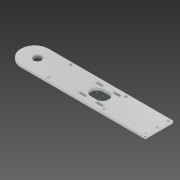
# Autodesk Inventor part: bovenarm - links
Saved by Autodesk Inventor 2020 (Build 240168000, 168)
## iProperties
Created: 2020-05-18
Part Number: bovenarm - links
Material: Generic
Document SubType Name: Modeling
Designer: stefa
Density: 1 g/cm^3
Appearance: Aluminum - Polished
Author: stefa
Autodesk Inventor part; units mm, degrees
ref_plane "YZ Plane" through (0, 0, 0) normal (1, 0, 0) x (0, 1, 0)
ref_plane "XZ Plane" through (0, 0, 0) normal (0, 1, 0) x (-1, 0, 0)
ref_plane "XY Plane" through (0, 0, 0) normal (0, 0, 1) x (1, 0, 0)
sketch "Sketch1" plane through (0, 0, 0) normal (0, 1, 0) x (-1, 0, 0)
  line L0 (0, 0) -> (250, 0)
  line L1 (250, 0) -> (250, -50)
  line L2 (250, -50) -> (0, -50)
  line L3 (0, -50) -> (0, 0)
  circle A0 centre (220, -25) radius 7
  line L4 (112.355, -25) -> (102.355, -25) construction
  line L5 (112.355, -13.9) -> (102.355, -13.9)
  line L6 (102.355, -36.1) -> (112.355, -36.1)
  arc A1 (112.355, -36.1) -> (112.355, -13.9) centre (112.355, -25) ccw
  arc A2 (102.355, -13.9) -> (102.355, -36.1) centre (102.355, -25) ccw
  line L7 (127.855, -40.5) -> (117.855, -40.5) construction
  line L8 (127.855, -38.95) -> (117.855, -38.95)
  line L9 (117.855, -42.05) -> (127.855, -42.05)
  arc A3 (127.855, -42.05) -> (127.855, -38.95) centre (127.855, -40.5) ccw
  arc A4 (117.855, -38.95) -> (117.855, -42.05) centre (117.855, -40.5) ccw
  line L10 (86.855, -42.05) -> (96.855, -42.05)
  arc A5 (96.855, -42.05) -> (96.855, -38.95) centre (96.855, -40.5) ccw
  line L11 (96.855, -40.5) -> (86.855, -40.5) construction
  line L12 (96.855, -38.95) -> (86.855, -38.95)
  arc A6 (86.855, -38.95) -> (86.855, -42.05) centre (86.855, -40.5) ccw
  line L13 (117.855, -11.05) -> (127.855, -11.05)
  arc A7 (127.855, -11.05) -> (127.855, -7.95) centre (127.855, -9.5) ccw
  line L14 (127.855, -9.5) -> (117.855, -9.5) construction
  line L15 (127.855, -7.95) -> (117.855, -7.95)
  arc A8 (117.855, -7.95) -> (117.855, -11.05) centre (117.855, -9.5) ccw
  line L16 (86.855, -11.05) -> (96.855, -11.05)
  arc A9 (96.855, -11.05) -> (96.855, -7.95) centre (96.855, -9.5) ccw
  line L17 (96.855, -9.5) -> (86.855, -9.5) construction
  line L18 (96.855, -7.95) -> (86.855, -7.95)
  arc A10 (86.855, -7.95) -> (86.855, -11.05) centre (86.855, -9.5) ccw
  circle A11 centre (180, -5) radius 2
  circle A12 centre (180, -45) radius 2
  circle A13 centre (80, -5) radius 2
  circle A14 centre (80, -45) radius 2
  circle A15 centre (4, -25) radius 2
  circle A16 centre (4, -45) radius 2
  circle A17 centre (4, -5) radius 2
  point P0 (107.355, -25)
  point P1 (122.855, -40.5)
  point P2 (91.855, -40.5)
  point P3 (122.855, -9.5)
  point P4 (91.855, -9.5)
  point P5 (0, -25)
  dimension "d0" = 250
  dimension "d1" = 50
  dimension "d16" = 14
  dimension "d18" = 25
  dimension "d24" = 22.2
  dimension "d25" = 3.1
  dimension "d26" = 10
  dimension "d27" = 10
  dimension "d28" = 112.645
  dimension "d29" = 25
  dimension "d30" = 30
  dimension "d31" = 15.5
  dimension "d32" = 15.5
  dimension "d35" = 31
  dimension "d38" = 31
  dimension "d42" = 4
  dimension "d43" = 70
  dimension "d44" = 5
  dimension "d47" = 40
  dimension "d50" = 100
  dimension "d53" = 4
  dimension "d54" = 4
  dimension "d55" = 20
  dimension "d56" = 20
  constraints: 48 end point, 20 point on circle, 18 centre point, 8 tangent, 5 parallel, 4 horizontal, 3 midpoint, 2 equal radius, 2 vertical, 2 vertical alignment, 1 horizontal alignment, 1 perpendicular, 42 other
  measures "d0" distance of L1.end L2.end
  measures "d1" distance of L0.end L1.end
  measures "d16" diameter of A0
  measures "d18" distance from line of L0 A0.centre
  measures "d24" diameter of A2
  measures "d25" diameter of A4
  measures "d26" distance of L9.start L9.end
  measures "d27" distance of L6.start L6.end
  measures "d28" distance of A0.centre point (107.355, -25)
  measures "d29" distance from line of L0 point (107.355, -25)
  measures "d30" distance from line of L1 A0.centre
  measures "d31" horizontal distance of point (107.355, -25) point (122.855, -40.5)
  measures "d32" horizontal distance of point (122.855, -40.5) point (107.355, -25)
  measures "d35" distance of L9.start L10.start
  measures "d38" distance of L9.start L13.start
  measures "d42" diameter of A11
  measures "d43" distance from line of L1 A11.centre
  measures "d44" distance from line of L0 A11.centre
  measures "d47" distance of A11.centre A12.centre
  measures "d50" distance of A11.centre A13.centre
  measures "d53" diameter of A15
  measures "d54" distance from line of L3 A15.centre
  measures "d55" distance of A17.centre A15.centre
  measures "d56" distance of A16.centre A15.centre
extrude "Extrusion1" add sketch "Sketch1" along normal blind 4
sketch "Sketch3" plane through (0, 4, 0) normal (0, 1, 0) x (1, 0, 0)
  line L0 (-123.455, 25) -> (-91.255, 25) construction
  arc A0 (-112.355, 36.1) -> (-112.355, 13.9) centre (-112.355, 25) ccw construction
  arc A1 (-102.355, 13.9) -> (-102.355, 36.1) centre (-102.355, 25) ccw construction
  point P0 (0, 0)
  constraints: 2 end point, 2 point on circle, 1 horizontal
fillet "Fillet1" radius 25 2 edges at (-250, 2, 0) (-250, 2, -50)
equation "\"d18\" = 0.5 * d1"
equation "\"d56\" = d55"
body "Solid1"
